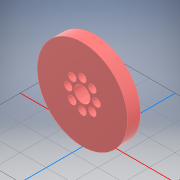
# Autodesk Inventor part: 000.005.004.003 - Поворотный диск
Saved by Autodesk Inventor 2022 (Build 260153000, 153)
## iProperties
Created: 2022-12-17
Part Number: 000.005.004.003 - Поворотный диск
Material: Пластик АБС
Document SubType Name: Modeling
Designer: Petrov Ivan
Density: 1.06 g/cm^3
Appearance: Гладкий — красный
Author: Petrov Ivan
Autodesk Inventor part; units mm, degrees
ref_plane "YZ Plane" through (0, 0, 0) normal (1, 0, 0) x (0, 1, 0)
ref_plane "XZ Plane" through (0, 0, 0) normal (0, 1, 0) x (-1, 0, 0)
ref_plane "XY Plane" through (0, 0, 0) normal (0, 0, 1) x (1, 0, 0)
sketch "Эскиз1" plane through (0, 0, 0) normal (0, 0, 1) x (1, 0, 0)
  circle A0 centre (0, 0) radius 14
  circle A1 centre (-11, 0) radius 1.2813
  circle A2 centre (-7.7782, -7.7782) radius 1.2813
  circle A3 centre (0, -11) radius 1.2813
  circle A4 centre (7.7782, -7.7782) radius 1.2813
  circle A5 centre (11, 0) radius 1.2813
  circle A6 centre (7.7782, 7.7782) radius 1.2813
  circle A7 centre (0, 11) radius 1.2813
  circle A8 centre (-7.7782, 7.7782) radius 1.2813
  circle A9 centre (0, 0) radius 6
  dimension "d3" = 12
  constraints: 10 centre point, 1 coincident
  measures "d3" diameter of A9
extrude "Выдавливание1" add sketch "Эскиз1" along normal blind 1.8
sketch "Эскиз2" plane through (0, 0, 1.8) normal (0, 0, 1) x (1, 0, 0)
  circle A0 centre (0, 0) radius 14 projected
  circle A1 centre (0, 0) radius 6 projected
  circle A2 centre (-7.7782, 7.7782) radius 1.2813 projected
  circle A3 centre (0, 11) radius 1.2813 projected
  circle A4 centre (7.7782, 7.7782) radius 1.2813 projected
  circle A5 centre (11, 0) radius 1.2813 projected
  circle A6 centre (7.7782, -7.7782) radius 1.2813 projected
  circle A7 centre (0, -11) radius 1.2813 projected
  circle A8 centre (-7.7782, -7.7782) radius 1.2813 projected
  circle A9 centre (-11, 0) radius 1.2813 projected
  circle A10 centre (0, 0) radius 35
  dimension "d4" = 70
  constraints: 1 centre point, 1 coincident
  measures "d4" diameter of A10
extrude "Выдавливание2" add sketch "Эскиз2" along normal blind 10 contours A0 | A10
sketch "Эскиз3" plane through (0, 0, 11.8) normal (0, 0, 1) x (1, 0, 0)
  circle A0 centre (0, 11) radius 1.2813 projected
  circle A1 centre (0, 11) radius 3
  point P0 (0, 0)
  dimension "d7" = 6
  constraints: 1 centre point, 1 coincident
  measures "d7" diameter of A1
extrude "Выдавливание3" cut sketch "Эскиз3" against normal blind 8
pattern_circular "Круговой массив1" count 8 over 360 about axis through (0, 0, 0) along (0, 0, 1) of "Выдавливание3"
